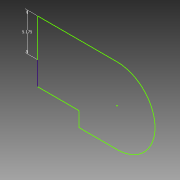
# Autodesk Inventor part: Lower Arm Bracket
Saved by Autodesk Inventor 2014 SP1 (Build 180222100, 222)
## iProperties
Created: 2013-12-29
Part Number: Lower Arm Bracket
Material: Generic
Document SubType Name: Modeling
Designer: tom
Density: 1 g/cm^3
Appearance: Default
Author: tom
Autodesk Inventor part; units mm, degrees
ref_plane "YZ Plane" through (0, 0, 0) normal (1, 0, 0) x (0, 1, 0)
ref_plane "XZ Plane" through (0, 0, 0) normal (0, 1, 0) x (-1, 0, 0)
ref_plane "XY Plane" through (0, 0, 0) normal (0, 0, 1) x (1, 0, 0)
sketch "Sketch1" plane through (0, 0, 0) normal (0, 0, 1) x (1, 0, 0)
  line L0 (0, 0) -> (0, -3.175)
  line L1 (0, -3.175) -> (5.66, -3.175)
  line L2 (0, 0) -> (0, 5.175)
  line L3 (0, 5.175) -> (10.835, 5.175)
  arc A0 (10.835, -5.175) -> (10.835, 5.175) centre (10.835, 0) ccw
  line L4 (10.835, -5.175) -> (5.66, -5.175)
  line L5 (5.66, -5.175) -> (5.66, -3.175)
  circle A1 centre (10.835, 0) radius 3.175
  dimension "d3" = 5.175
  dimension "d4" = 6.35
  constraints: 12 end point, 3 perpendicular, 2 centre point, 2 point on circle, 1 coincident, 1 parallel, 1 tangent, 1 vertical
  measures "d3" distance of L0.start L2.end
  measures "d4" diameter of A1
extrude "Extrusion1" add sketch "Sketch1" along normal blind 5.66
body "Solid1"
